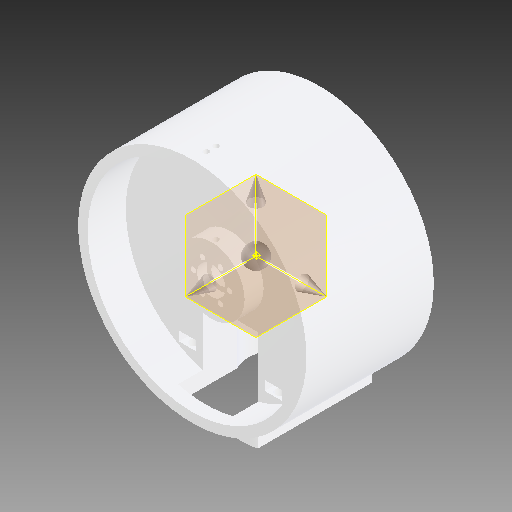
# Autodesk Inventor part: AA035
Saved by Autodesk Inventor 2017 SP1 (Build 210196100, 196)
## iProperties
Created: 2017-10-23
Part Number: AA035
Material: ABS Plastic
Document SubType Name: Modeling
Designer: Zach
Categories: <?xml version="1.0" encoding="UTF-16"?> <MemberInstance><Categories><FamilyTemplate><FamilyTemplateParameter ValueType="xs:double" Id="1" ObjectReferenceKey="da_z" ObjectType="kUserParameterObject"/><FamilyTemplateParameter ValueType="xs:double" Id="2" ObjectReferenceKey="da_b" ObjectType="kUserParameterObject"/><FamilyTemplateParameter ValueType="xs:double" Id="3" ObjectReferenceKey="da_beta" ObjectType="kUserParameterObject"/><FamilyTemplateParameter ValueType="xs:double" Id="4" ObjectReferenceKey="da_da" ObjectType="kUserParameterObject"/><FamilyTemplateParameter ValueType="xs:double" Id="5" ObjectReferenceKey="da_aw" ObjectType="kUserParameterObject"/><FamilyTemplateParameter ValueType="xs:string" Id="6" ObjectReferenceKey="EAIAABAAAACIAQAAAAAAAIAAAAAAAAAA" ObjectType="83910656" SubObjectId="SurfaceGeometry"/></FamilyTemplate><ParamToTemplateMap><ParamToTemplate CategoryParameter="//CategoryParameter[@InternalName='046C89C9-8512-4d59-83FE-43B91F4F132A']" TemplateParameter="1"/><ParamToTemplate CategoryParameter="//CategoryParameter[@InternalName='2552DF32-E462-4b46-AEBF-C6C7768E72AC']" TemplateParameter="2"/><ParamToTemplate CategoryParameter="//CategoryParameter[@InternalName='C9EE641D-15FC-4fae-A226-E94C4372FDD7']" TemplateParameter="3"/><ParamToTemplate><ParamToTemplate CategoryParameter="//CategoryParameter[@InternalName='00B6519A-459B-49c7-AD84-2E56D39A5744']" ConstantValue="0.341447"/></ParamToTemplate><ParamToTemplate><ParamToTemplate CategoryParameter="//CategoryParameter[@InternalName='04B31F0E-C7A6-4894-AA32-9629BEFACF47']" ConstantValue="1.000000"/></ParamToTemplate><ParamToTemplate><ParamToTemplate CategoryParameter="//CategoryParameter[@InternalName='43CBEC2E-7847-49e7-A936-2F7889FCB2D9']" ConstantValue="0.250000"/></ParamToTemplate><ParamToTemplate><ParamToTemplate CategoryParameter="//CategoryParameter[@InternalName='B1EFC894-105D-4ebd-86BF-FA20ED196853']" ConstantValue="0.350000"/></ParamToTemplate><ParamToTemplate><ParamToTemplate CategoryParameter="//CategoryParameter[@InternalName='51175063-3D10-4879-93E8-6246FE8B403D']" ConstantValue="2060000000.000000"/></ParamToTemplate><ParamToTemplate><ParamToTemplate CategoryParameter="//CategoryParameter[@InternalName='A3A52E27-4454-46a9-B0BD-C932399B70AF']" ConstantValue="0.300000"/></ParamToTemplate><ParamToTemplate><ParamToTemplate CategoryParameter="//CategoryParameter[@InternalName='91B76062-C214-41d9-B1B9-14D2AB99603D']" ConstantValue="0.200000"/></ParamToTemplate><ParamToTemplate><ParamToTemplate CategoryParameter="//CategoryParameter[@InternalName='374E806E-8B8A-4dda-A9AA-1039D6500AD2']" ConstantValue="5.000000"/></ParamToTemplate><ParamToTemplate><ParamToTemplate CategoryParameter="//CategoryParameter[@InternalName='2D373A89-B862-43d6-8D0B-0CBF12AB9F6C']" ConstantValue="0.392699"/></ParamToTemplate><ParamToTemplate CategoryParameter="//CategoryParameter[@InternalName='37777632-D6A2-4fac-9D53-DB8ACD95C989']" TemplateParameter="4"/><ParamToTemplate CategoryParameter="//CategoryParameter[@InternalName='FD1017F1-B727-4f7e-9707-0F86F1FF9423']" TemplateParameter="5"/><ParamToTemplate><ParamToTemplate CategoryParameter="//CategoryParameter[@InternalName='9E1B4470-B2D3-4ff1-B813-535BB4CDF51A']" ConstantValue="3520000.000000"/></ParamToTemplate><ParamToTemplate><ParamToTemplate CategoryParameter="//CategoryParameter[@InternalName='F8452263-BFF6-458c-9FB1-07C4B99E95CD']" ConstantValue="11400000.000000"/></ParamToTemplate><ParamToTemplate><ParamToTemplate CategoryParameter="//CategoryParameter[@InternalName='3E3BB259-FD49-497f-8171-6EBC954A3479']" ConstantValue="2.000000"/></ParamToTemplate><ParamToTemplate CategoryParameter="//CategoryParameter[@InternalName='27C3BAF2-7550-4e4b-AE2C-0DB134B7D9B7']" TemplateParameter="6"/></ParamToTemplateMap><Category DisplayName="Gear" InternalName="DC85795E-93AB-48d5-8EEE-5A27447B64BD" Mnemonic="Gear"><CategoryParameter DisplayName="z" InternalName="046C89C9-8512-4d59-83FE-43B91F4F132A" Mnemonic="z"/><CategoryParameter DisplayName="b" InternalName="2552DF32-E462-4b46-AEBF-C6C7768E72AC" Mnemonic="b"/><CategoryParameter DisplayName="||b|" InternalName="C9EE641D-15FC-4fae-A226-E94C4372FDD7" Mnemonic="beta"/><CategoryParameter DisplayName="x" InternalName="00B6519A-459B-49c7-AD84-2E56D39A5744" Mnemonic="x"/><CategoryParameter DisplayName="a*" InternalName="04B31F0E-C7A6-4894-AA32-9629BEFACF47" Mnemonic="a"/><CategoryParameter DisplayName="c*" InternalName="43CBEC2E-7847-49e7-A936-2F7889FCB2D9" Mnemonic="c"/><CategoryParameter DisplayName="r|.f|*" InternalName="B1EFC894-105D-4ebd-86BF-FA20ED196853" Mnemonic="rf"/><CategoryParameter DisplayName="E" InternalName="51175063-3D10-4879-93E8-6246FE8B403D" Mnemonic="E"/><CategoryParameter DisplayName="||m|" InternalName="A3A52E27-4454-46a9-B0BD-C932399B70AF" Mnemonic="mi"/><Category DisplayName="SpurGear" InternalName="26C5A22E-A91E-4dfd-A3B3-23CCAFAE1764" Mnemonic="SpurGear"><CategoryParameter DisplayName="m" InternalName="91B76062-C214-41d9-B1B9-14D2AB99603D" Mnemonic="m"/><CategoryParameter DisplayName="P" InternalName="374E806E-8B8A-4dda-A9AA-1039D6500AD2" Mnemonic="PP"/><CategoryParameter DisplayName="||a|" InternalName="2D373A89-B862-43d6-8D0B-0CBF12AB9F6C" Mnemonic="alpha"/><CategoryParameter DisplayName="d|.a|" InternalName="37777632-D6A2-4fac-9D53-DB8ACD95C989" Mnemonic="da"/><CategoryParameter DisplayName="a|.w|" InternalName="FD1017F1-B727-4f7e-9707-0F86F1FF9423" Mnemonic="aw"/><CategoryParameter DisplayName="||s||.Flim|" InternalName="9E1B4470-B2D3-4ff1-B813-535BB4CDF51A" Mnemonic="sFlim"/><CategoryParameter DisplayName="||s||.Hlim|" InternalName="F8452263-BFF6-458c-9FB1-07C4B99E95CD" Mnemonic="sHlim"/><CategoryParameter DisplayName="type" InternalName="3E3BB259-FD49-497f-8171-6EBC954A3479" Mnemonic="type"/><CategoryParameter DisplayName="PitchDiameter" InternalName="27C3BAF2-7550-4e4b-AE2C-0DB134B7D9B7" Mnemonic="IDS_PITCHDIAM"/></Category></Category></Categories></MemberInstance>
Density: 1.06 g/cm^3
Appearance: CR White
CustomPartVersion: 1
Author: Zach
Title: AA035.ipt
Autodesk Inventor part; units mm, degrees
ref_plane "YZ Plane" through (0, 0, 0) normal (1, 0, 0) x (0, 1, 0)
sketch "Sketch3" plane through (0, 0, 0) normal (0, 0, 1) x (1, 0, 0)
  circle A0 centre (0, 0) radius 60
  dimension "d49" = 120
  constraints: 1 centre point, 1 coincident
  measures "d49" diameter of A0
sketch "Sketch3 outline for Extrusion2" plane through (0, 0, 0) normal (0, 0, 1) x (1, 0, 0)
  circle A0 centre (0, 0) radius 60
extrude "Extrusion2" add sketch "Sketch3 outline for Extrusion2" along normal blind 67
sketch "Sketch4" plane through (0, 0, 0) normal (0, 0, -1) x (-1, 0, 0)
  circle A0 centre (0, 0) radius 5
  dimension "d52" = 10
  constraints: 1 centre point, 1 coincident
  measures "d52" diameter of A0
sketch "Sketch4 outline for Extrusion3" plane through (0, 0, 0) normal (0, 0, -1) x (-1, 0, 0)
  circle A0 centre (0, 0) radius 5
extrude "Extrusion3" cut sketch "Sketch4 outline for Extrusion3" against normal through all
ref_plane "Work Plane11" through (0, 0, 46) normal (0, 0, 1) x (1, 0, 0)
sketch "Sketch6" plane through (0, 0, 46) normal (0, 0, 1) x (1, 0, 0)
  line L0 (-27.5, -53.326823) -> (27.5, -53.326823)
  line L1 (27.5, -53.326823) -> (27.5, -61.326823)
  line L2 (27.5, -61.326823) -> (-27.5, -61.326823)
  line L3 (-27.5, -61.326823) -> (-27.5, -53.326823)
  circle A0 centre (0, 0) radius 5 construction
  circle A1 centre (0, 0) radius 60 construction
  dimension "d63" = 55
  dimension "d64" = 8
  constraints: 8 end point, 2 parallel, 2 point on circle, 1 horizontal, 1 perpendicular
  measures "d63" distance of L1.end L2.end
  measures "d64" distance of L0.end L1.end
sketch "Sketch6 outline for Extrusion5" plane through (0, 0, 46) normal (0, 0, 1) x (1, 0, 0)
  line L0 (-27.5, -53.326823) -> (27.5, -53.326823)
  line L1 (27.5, -53.326823) -> (27.5, -61.326823)
  line L2 (27.5, -61.326823) -> (-27.5, -61.326823)
  line L3 (-27.5, -61.326823) -> (-27.5, -53.326823)
extrude "Extrusion5" add sketch "Sketch6 outline for Extrusion5" along normal mid plane 42
sketch "Sketch7" plane through (0, 0, 46) normal (0, 0, 1) x (1, 0, 0)
  line L0 (-41, -61.326823) -> (41, -61.326823)
  line L1 (41.521509, -76.326823) -> (-41.521509, -76.326823)
  line L2 (27.5, -61.326823) -> (-27.5, -61.326823)
  line L3 (-41.521509, -76.326823) -> (-41, -61.326823)
  line L4 (41.521509, -76.326823) -> (41, -61.326823)
  point P0 (0, 0)
  point P1 (0, -61.326823)
  point P2 (0, -76.326823)
  dimension "d67" = 83.04302
  dimension "d99" = 82
  dimension "d100" = 15
  constraints: 8 end point, 3 midpoint, 1 horizontal, 1 parallel, 1 vertical alignment
  measures "d67" distance of L1.start L1.end
  measures "d99" distance of L0.start L0.end
  measures "d100" distance between parallel lines of L0 L1
sketch "Sketch7 outline for Extrusion6" plane through (0, 0, 46) normal (0, 0, 1) x (1, 0, 0)
  line L0 (-41, -61.326823) -> (0, -61.326823)
  line L1 (0, -61.326823) -> (41, -61.326823)
  line L2 (41, -61.326823) -> (41.521509, -76.326823)
  line L3 (41.521509, -76.326823) -> (-41.521509, -76.326823)
  line L4 (-41.521509, -76.326823) -> (-41, -61.326823)
extrude "Extrusion6" add sketch "Sketch7 outline for Extrusion6" along normal mid plane 80
sketch "Sketch8" plane through (-41.521509, -76.326823, 86) normal (0, -1, 0) x (1, 0, 0)
  line L0 (64.021509, -62.5) -> (19.021509, -62.5) construction
  line L1 (19.021509, -62.5) -> (19.021509, -17.5) construction
  line L2 (19.021509, -17.5) -> (64.021509, -17.5) construction
  line L3 (64.021509, -17.5) -> (64.021509, -62.5) construction
  circle A0 centre (64.021509, -62.5) radius 2.5
  circle A1 centre (64.021509, -17.5) radius 2.5
  circle A2 centre (19.021509, -62.5) radius 2.5
  circle A3 centre (19.021509, -17.5) radius 2.5
  line L4 (0, 0) -> (83.043018, 0)
  line L5 (83.043018, 0) -> (83.043018, -80)
  point P0 (23.25, -86)
  point P1 (41.521509, -17.5)
  point P2 (41.521509, 0)
  point P3 (83.043018, -40)
  dimension "d75" = 45
  dimension "d78" = 5
  dimension "d79" = 5
  dimension "d101" = 45
  dimension "d102" = 5
  dimension "d103" = 5
  dimension "d184" = 17.5
  constraints: 8 end point, 4 centre point, 4 coincident, 3 midpoint, 2 parallel, 1 horizontal, 1 perpendicular, 1 vertical alignment
  measures "d75" distance of L0.end L1.end
  measures "d78" diameter of A2
  measures "d79" diameter of A3
  measures "d101" distance of L1.end L2.end
  measures "d102" diameter of A1
  measures "d103" diameter of A0
  measures "d184" distance between parallel lines of L4 L2
sketch "Sketch8 outline for Extrusion7" plane through (-41.521509, -76.326823, 86) normal (0, -1, 0) x (1, 0, 0)
  circle A0 centre (64.021509, -17.5) radius 2.5
  circle A1 centre (19.021509, -17.5) radius 2.5
extrude "Extrusion7" cut sketch "Sketch8 outline for Extrusion7" against normal blind 25
sketch "Sketch9" plane through (-41.521509, -76.326823, 86) normal (0, -1, 0) x (1, 0, 0)
  circle A0 centre (41.521509, -40) radius 16.5
  circle A1 centre (64.021509, -17.5) radius 2.5 construction
  circle A2 centre (19.021509, -17.5) radius 2.5 construction
  line L0 (83.043018, 0) -> (83.043018, -80) construction
  line L1 (0, 0) -> (83.043018, 0) construction
  line L2 (0, 0) -> (0, -80) construction
  line L3 (83.043018, -80) -> (0, -80) construction
  point P0 (23.25, -86)
  point P1 (0, -40)
  point P2 (41.521509, 0)
  dimension "d82" = 33
  constraints: 2 midpoint, 1 centre point, 1 horizontal alignment, 1 vertical alignment
  measures "d82" diameter of A0
sketch "Sketch9 outline for Extrusion8" plane through (-41.521509, -76.326823, 86) normal (0, -1, 0) x (1, 0, 0)
  circle A0 centre (41.521509, -40) radius 16.5
extrude "Extrusion8" cut sketch "Sketch9 outline for Extrusion8" against normal blind 45
sketch "Sketch14" plane through (0, 0, 46) normal (0, 0, 1) x (1, 0, 0)
  line L0 (16.5, -76.326823) -> (16.5, -31.326823)
  line L1 (16.5, -31.326823) -> (-16.5, -31.326823)
  line L2 (-16.5, -31.326823) -> (-16.5, -16.326823)
  line L3 (-16.5, -16.326823) -> (16.5, -16.326823)
  line L4 (16.5, -16.326823) -> (16.5, -31.326823)
  point P0 (0, 0)
  dimension "d91" = 33
  dimension "d92" = 15
  constraints: 8 end point, 2 parallel, 1 horizontal, 1 perpendicular
  measures "d91" distance of L2.end L3.end
  measures "d92" distance of L1.end L2.end
sketch "Sketch14 outline for Extrusion10" plane through (0, 0, 46) normal (0, 0, 1) x (1, 0, 0)
  line L0 (16.5, -31.326823) -> (-16.5, -31.326823)
  line L1 (-16.5, -31.326823) -> (-16.5, -16.326823)
  line L2 (-16.5, -16.326823) -> (16.5, -16.326823)
  line L3 (16.5, -16.326823) -> (16.5, -31.326823)
extrude "Extrusion10" cut sketch "Sketch14 outline for Extrusion10" along normal mid plane 33
fillet "Fillet4" radius 20 4 edges at (41.2608, -68.8268, 86) (41.2608, -68.8268, 6) (-41.2608, -68.8268, 86) (-41.2608, -68.8268, 6)
ref_plane "Work Plane15" through (0, 0, 25) normal (0, 0, -1) x (-0.9685832, -0.2486899, 0)
sketch "Sketch16" plane through (0, 0, 25) normal (0, 0, -1) x (-0.9685832, -0.2486899, 0)
  circle A0 centre (0, 0) radius 60
  circle A1 centre (0, 0) radius 63
  dimension "d107" = 3
  constraints: 2 centre point
  measures "d107" radial gap between concentric circles of A0 A1
sketch "Sketch16 outline for Extrusion12" plane through (0, 0, 25) normal (0, 0, -1) x (-0.9685832, -0.2486899, 0)
  circle A0 centre (0, 0) radius 63
extrude "Extrusion12" cut sketch "Sketch16 outline for Extrusion12" along normal through all
sketch "Sketch17" plane through (0, 0, 25) normal (0, 0, -1) x (-1, 0, 0)
  circle A0 centre (33.807404, 9.058667) radius 2.5
  circle A1 centre (9.058667, 33.807404) radius 2.5
  circle A2 centre (-24.748737, 24.748737) radius 2.5
  circle A3 centre (-33.807404, -9.058667) radius 2.5
  circle A4 centre (-9.058667, -33.807404) radius 2.5
  circle A5 centre (24.748737, -24.748737) radius 2.5
  line L0 (33.807404, 9.058667) -> (-33.807404, -9.058667) construction
  line L1 (-1.798057, -79.48798) -> (39.754961, -68.353883)
  line L2 (0, 0) -> (32.565454, 0)
  circle A6 centre (0, 0) radius 5
  line L3 (14.422928, -61.326823) -> (27.5, -61.326823)
  line L4 (27.5, -61.326823) -> (27.5, -53.326823)
  arc A7 (27.5, -53.326823) -> (-27.5, -53.326823) centre (0, 0) ccw
  line L5 (-27.5, -53.326823) -> (-27.5, -61.326823)
  line L6 (-27.5, -61.326823) -> (-14.422928, -61.326823)
  arc A8 (-14.422928, -61.326823) -> (14.422928, -61.326823) centre (0, 0) ccw
  dimension "d108" = 5
  dimension "d109" = 35
  dimension "d112" = 360
  dimension "d207" = 15
  constraints: 6 centre point, 6 end point, 1 coincident, 1 horizontal, 1 midpoint, 1 parallel, 13 other
  measures "d108" diameter of A0
  measures "d109" distance of L2.start L0.start
  measures "d207" angle of L0 L2
sketch "Sketch17 outline for Extrusion13" plane through (0, 0, 25) normal (0, 0, -1) x (-1, 0, 0)
  circle A0 centre (33.807404, 9.058667) radius 2.5
  circle A1 centre (9.058667, 33.807404) radius 2.5
  circle A2 centre (-24.748737, 24.748737) radius 2.5
  circle A3 centre (-33.807404, -9.058667) radius 2.5
extrude "Extrusion13" cut sketch "Sketch17 outline for Extrusion13" against normal blind 25
sketch "Sketch20" plane through (0, 0, 67) normal (0, 0, 1) x (1, 0, 0)
  arc A0 (27.5, -53.326823) -> (-27.5, -53.326823) centre (0, 0) ccw
  circle A1 centre (0, 0) radius 60
  circle A2 centre (0, 0) radius 5
  constraints: 1 coincident, 3 other
sketch "Sketch20 outline for Extrusion15" plane through (0, 0, 67) normal (0, 0, 1) x (1, 0, 0)
  circle A0 centre (0, 0) radius 60
  circle A1 centre (0, 0) radius 5
extrude "Extrusion15" add sketch "Sketch20 outline for Extrusion15" along normal blind 25
sketch "Sketch21" plane through (-21.509425, -76.326823, 6) normal (0, -1, 0) x (1, 0, 0)
  line L0 (36.009425, 79) -> (7.009425, 79)
  line L1 (7.009425, 79) -> (7.009425, 55)
  line L2 (7.009425, 55) -> (36.009425, 55)
  line L3 (36.009425, 55) -> (36.009425, 79)
  circle A0 centre (21.509425, 40) radius 16.5
  line L4 (36.009425, 67) -> (7.009425, 67)
  point P0 (21.509425, -6)
  point P1 (21.509425, 67)
  dimension "d124" = 29
  dimension "d125" = 24
  dimension "d126" = 27
  constraints: 10 end point, 3 midpoint, 2 parallel, 1 horizontal, 1 perpendicular, 1 vertical alignment
  measures "d124" distance of L2.end L1.end
  measures "d125" distance of L1.end L0.end
  measures "d126" distance from line of L4 A0.centre
sketch "Sketch21 outline for Extrusion16" plane through (-21.509425, -76.326823, 6) normal (0, -1, 0) x (1, 0, 0)
  line L0 (7.009425, 55) -> (36.009425, 55)
  line L1 (36.009425, 55) -> (36.009425, 79)
  line L2 (36.009425, 79) -> (7.009425, 79)
  line L3 (7.009425, 79) -> (7.009425, 55)
extrude "Extrusion16" cut sketch "Sketch21 outline for Extrusion16" against normal blind 15
sketch "Sketch22" plane through (-27.5, -61.326823, 67) normal (0, 1, 0) x (1, 0, 0)
  line L0 (55, 0) -> (55, 42)
  line L1 (0, 0) -> (0, 42)
  line L2 (0, 0) -> (3, 0)
  line L3 (55, 0) -> (55, -17.911477)
  line L4 (0, 0) -> (0, -17.911477)
  line L5 (5.990575, -19) -> (6.512084, -19) construction
  line L6 (-13.5, 1) -> (-14.021509, 1) construction
  circle A0 centre (5, -1.5) radius 2.5
  line L7 (42, -18) -> (42, 6)
  line L8 (13, -18) -> (42, -18)
  line L9 (13, 6) -> (13, -18)
  line L10 (7, 0) -> (13, 0)
  line L11 (13, 0) -> (13, -18)
  line L12 (13, -18) -> (42, -18)
  line L13 (55, 0) -> (52, 0)
  circle A1 centre (50, -1.5) radius 2.5
  line L14 (48, 0) -> (42, 0)
  line L15 (42, 0) -> (42, -18)
  arc A2 (48, 0) -> (52, 0) centre (50, -1.5) ccw
  arc A3 (3, 0) -> (7, 0) centre (5, -1.5) ccw
  line L16 (5.990575, -19) -> (6.285813, -19)
  line L17 (-13.5, 1) -> (-14.021509, 1)
  line L18 (5.990575, -19) -> (6.512084, -19)
  line L19 (48.487916, -19) -> (49.009425, -19)
  arc A4 (0, -17.911477) -> (6.285813, -19) centre (6.512084, 1) ccw
  arc A5 (48.487916, -19) -> (55, -17.911477) centre (48.487997, 1.023032) ccw
  line L20 (48.487916, -19) -> (6.285813, -19)
  line L21 (5.990575, -19) -> (49.009425, -19)
  ellipse E0 centre (5.990575, 1) end of major axis (-14.021509, 1) minor radius 20 (-14.021509, 1) -> (5.990575, -19) ccw
  line L22 (5.990575, -19) -> (6.512084, -19)
  ellipse E1 centre (6.512084, 1) end of major axis (-13.5, 1) minor radius 20 (-13.5, 1) -> (6.512084, -19) ccw
  line L23 (-13.5, 1) -> (-14.021509, 1)
  ellipse E2 centre (48.487916, 1) end of major axis (68.5, 1) minor radius 20 (48.487916, -19) -> (68.5, 1) ccw
  line L24 (48.487916, -19) -> (49.009425, -19)
  ellipse E3 centre (49.009425, 1) end of major axis (69.021509, 1) minor radius 20 (49.009425, -19) -> (69.021509, 1) ccw
  line L25 (69.021509, 1) -> (68.5, 1)
  point P0 (27.5, 67)
  point P1 (51.789134, -18.726001)
  constraints: 22 end point, 11 point on circle, 4 centre point, 4 point on line, 3 perpendicular, 2 coincident, 2 collinear, 2 vertical, 1 horizontal, 1 horizontal alignment, 10 other
sketch "Sketch22 outline for Extrusion17" plane through (-27.5, -61.326823, 67) normal (0, 1, 0) x (1, 0, 0)
  line L0 (55, -17.911477) -> (55, 0)
  arc A0 (51.789134, -18.726001) -> (55, -17.911477) centre (48.487997, 1.023032) ccw
  arc A1 (48.487916, -19) -> (51.789134, -18.726001) centre (48.487997, 1.023032) ccw
  line L1 (6.285813, -19) -> (48.487916, -19)
  arc A2 (0, -17.911477) -> (6.285813, -19) centre (6.512084, 1) ccw
  line L2 (0, 0) -> (0, -17.911477)
  line L3 (3, 0) -> (0, 0)
  arc A3 (7, 0) -> (3, 0) centre (5, -1.5) cw
  line L4 (13, 0) -> (7, 0)
  line L5 (13, -18) -> (13, 0)
  line L6 (42, -18) -> (13, -18)
  line L7 (42, 0) -> (42, -18)
  line L8 (48, 0) -> (42, 0)
  arc A4 (52, 0) -> (48, 0) centre (50, -1.5) cw
  line L9 (55, 0) -> (52, 0)
extrude "Extrusion17" add sketch "Sketch22 outline for Extrusion17" along normal blind 15
sketch "Sketch23" plane through (-21.509425, -76.326823, 6) normal (0, -1, 0) x (1, 0, 0)
  line L0 (36.009425, 79) -> (36.009425, 55)
  line L1 (36.009425, 55) -> (7.009425, 55)
  line L2 (7.009425, 55) -> (7.009425, 79)
  line L3 (7.009425, 79) -> (36.009425, 79)
  point P0 (21.509425, -6)
sketch "Sketch23 outline for Extrusion18" plane through (-21.509425, -76.326823, 6) normal (0, -1, 0) x (1, 0, 0)
  line L0 (36.009425, 79) -> (36.009425, 55)
  line L1 (36.009425, 55) -> (7.009425, 55)
  line L2 (7.009425, 55) -> (7.009425, 79)
  line L3 (7.009425, 79) -> (36.009425, 79)
extrude "Extrusion18" cut sketch "Sketch23 outline for Extrusion18" against normal blind 20
sketch "Sketch25" plane through (-21.509425, -56.326823, 6) normal (0, -1, 0) x (1, 0, 0)
  line L0 (36.009425, 55) -> (28.383288, 55)
  arc A0 (21.509425, 56.5) -> (5.009425, 40) centre (21.509425, 40) ccw
  line L1 (36.009425, 55) -> (7.009425, 55)
  line L2 (7.009425, 55) -> (7.009425, 47.874008)
  line L3 (7.009425, 47.874008) -> (36.009425, 47.874008)
  line L4 (36.009425, 47.874008) -> (36.009425, 55)
  point P0 (21.509425, -6)
  constraints: 8 end point, 2 parallel, 1 horizontal, 1 perpendicular, 1 point on circle, 1 vertical alignment
sketch "Sketch25 outline for Extrusion20" plane through (-21.509425, -56.326823, 6) normal (0, -1, 0) x (1, 0, 0)
  line L0 (36.009425, 47.874008) -> (36.009425, 55)
  line L1 (7.009425, 47.874008) -> (36.009425, 47.874008)
  line L2 (7.009425, 55) -> (7.009425, 47.874008)
  line L3 (36.009425, 55) -> (7.009425, 55)
extrude "Extrusion20" cut sketch "Sketch25 outline for Extrusion20" along normal blind 25
sketch "Sketch26" plane through (0, 0, 92) normal (0, 0, 1) x (1, 0, 0)
  circle A0 centre (0, 0) radius 5 projected
  circle A1 centre (0, 0) radius 13.5
  dimension "d138" = 27
  constraints: 1 centre point, 1 coincident
  measures "d138" diameter of A1
sketch "Sketch26 outline for Extrusion21" plane through (0, 0, 92) normal (0, 0, 1) x (1, 0, 0)
  circle A0 centre (0, 0) radius 13.5
  circle A1 centre (0, 0) radius 5
extrude "Extrusion21" cut sketch "Sketch26 outline for Extrusion21" against normal blind 10
sketch "Sketch27" plane through (0, 0, 82) normal (0, 0, 1) x (1, 0, 0)
  circle A0 centre (9.525, 0) radius 1.5
  circle A1 centre (4.7625, 8.248892) radius 1.5
  circle A2 centre (-4.7625, 8.248892) radius 1.5
  circle A3 centre (-9.525, 0) radius 1.5
  circle A4 centre (-4.7625, -8.248892) radius 1.5
  circle A5 centre (4.7625, -8.248892) radius 1.5
  point P0 (0, 0)
  dimension "d141" = 3
  dimension "d142" = 9.525
  dimension "d145" = 360
  constraints: 6 centre point, 1 horizontal alignment, 13 other
  measures "d141" diameter of A0
  measures "d142" distance of point (0, 0) A0.centre
sketch "Sketch27 outline for Extrusion22" plane through (0, 0, 82) normal (0, 0, 1) x (1, 0, 0)
  circle A0 centre (9.525, 0) radius 1.5
  circle A1 centre (4.7625, 8.248892) radius 1.5
  circle A2 centre (-4.7625, 8.248892) radius 1.5
  circle A3 centre (-9.525, 0) radius 1.5
  circle A4 centre (-4.7625, -8.248892) radius 1.5
  circle A5 centre (4.7625, -8.248892) radius 1.5
extrude "Extrusion22" cut sketch "Sketch27 outline for Extrusion22" against normal blind 15
sketch "Sketch28" plane through (0, 0, 0) normal (0, 1, 0) x (-1, 0, 0)
  circle A0 centre (0, 79.65) radius 1.5
  circle A1 centre (0, 84.75) radius 1.5
  line L0 (5, 82) -> (-5, 82) projected
  line L1 (0, 82) -> (0, 83.25)
  line L2 (0, 83.25) -> (0, 81.15)
  point P0 (0, 0)
  point P1 (0, 86.25)
  dimension "d151" = 3
  dimension "d150" = 3
  dimension "d153" = 1.25
  dimension "d166" = 2.1
  constraints: 4 end point, 4 vertical alignment, 2 point on circle, 2 vertical, 1 centre point, 1 midpoint, 2 other
  measures "d150" diameter of A1
  measures "d153" distance of L1.start L1.end
  measures "d166" distance of L1.end L2.end
sketch "Sketch28 outline for Extrusion23" plane through (0, 0, 0) normal (0, 1, 0) x (-1, 0, 0)
  circle A0 centre (0, 79.65) radius 1.5
  circle A1 centre (0, 84.75) radius 1.5
extrude "Extrusion23" cut sketch "Sketch28 outline for Extrusion23" along normal through all
sketch "Sketch29" plane through (0, 0, 92) normal (0, 0, 1) x (1, 0, 0)
  circle A0 centre (0, 0) radius 17.5
  circle A1 centre (0, 0) radius 55
  circle A2 centre (0, 0) radius 60 construction
  dimension "d156" = 35
  dimension "d179" = 5
  constraints: 2 centre point, 2 coincident
  measures "d156" diameter of A0
  measures "d179" radial gap between concentric circles of A1 A2
sketch "Sketch29 outline for Extrusion24" plane through (0, 0, 92) normal (0, 0, 1) x (1, 0, 0)
  circle A0 centre (0, 0) radius 55
  circle A1 centre (0, 0) radius 17.5
extrude "Extrusion24" cut sketch "Sketch29 outline for Extrusion24" against normal blind 20
sketch "Sketch30" plane through (0, 0, 82) normal (0, 0, 1) x (1, 0, 0)
  circle A0 centre (0, 0) radius 17.5 projected
sketch "Sketch30 outline for Extrusion25" plane through (0, 0, 82) normal (0, 0, 1) x (1, 0, 0)
  circle A0 centre (0, 0) radius 17.5
extrude "Extrusion25" cut sketch "Sketch30 outline for Extrusion25" along normal through all
sketch "Sketch32" plane through (0, 0, 82) normal (0, 0, 1) x (1, 0, 0)
  circle A0 centre (0, 0) radius 7.5
  dimension "d162" = 15
  constraints: 1 centre point, 1 coincident
  measures "d162" diameter of A0
sketch "Sketch32 outline for Extrusion26" plane through (0, 0, 82) normal (0, 0, 1) x (1, 0, 0)
  circle A0 centre (0, 0) radius 7.5
extrude "Extrusion26" cut sketch "Sketch32 outline for Extrusion26" against normal blind 5
sketch "Sketch34" plane through (0, 0, 72) normal (0, 0, 1) x (1, 0, 0)
  line L0 (-14.5, -56.326823) -> (-14.5, -76.326823)
  line L1 (-14.5, -56.326823) -> (14.5, -56.326823)
  line L2 (14.5, -56.326823) -> (14.5, -21.326823)
  line L3 (14.5, -21.326823) -> (-14.5, -21.326823)
  line L4 (-14.5, -21.326823) -> (-14.5, -56.326823)
  line L5 (14.5, -76.326823) -> (14.5, -56.326823)
  point P0 (0, 0)
  dimension "d167" = 35
  constraints: 8 end point, 2 parallel, 1 coincident, 1 horizontal, 1 perpendicular
  measures "d167" distance of L1.end L2.end
sketch "Sketch34 outline for Extrusion27" plane through (0, 0, 72) normal (0, 0, 1) x (1, 0, 0)
  line L0 (-14.5, -21.326823) -> (-14.5, -56.326823)
  line L1 (14.5, -21.326823) -> (-14.5, -21.326823)
  line L2 (14.5, -56.326823) -> (14.5, -21.326823)
  line L3 (-14.5, -56.326823) -> (14.5, -56.326823)
extrude "Extrusion27" cut sketch "Sketch34 outline for Extrusion27" along normal blind 13 and the other way blind 20
sketch "Sketch35" plane through (41, -61.326823, 66) normal (0, 1, 0) x (1, 0, 0)
  line L0 (-109.517427, 73.180887) -> (100.55897, 73.180887)
  line L1 (100.55897, 73.180887) -> (100.55897, -75.26578)
  line L2 (100.55897, -75.26578) -> (-109.517427, -75.26578)
  line L3 (-109.517427, -75.26578) -> (-109.517427, 73.180887)
  point P0 (-22.5, 23.5)
  constraints: 8 end point, 2 parallel, 1 horizontal, 1 perpendicular
sketch "Sketch35 outline for Extrusion28" plane through (41, -61.326823, 66) normal (0, 1, 0) x (1, 0, 0)
  line L0 (-109.517427, 73.180887) -> (100.55897, 73.180887)
  line L1 (100.55897, 73.180887) -> (100.55897, -75.26578)
  line L2 (100.55897, -75.26578) -> (-109.517427, -75.26578)
  line L3 (-109.517427, -75.26578) -> (-109.517427, 73.180887)
extrude "Extrusion28" cut sketch "Sketch35 outline for Extrusion28" against normal through all
sketch "Sketch37" plane through (0, 0, 92) normal (0, 0, 1) x (1, 0, 0)
  line L0 (-60, 14.5) -> (-53.054218, 14.5)
  line L1 (-53.054218, 14.5) -> (-53.054218, -14.5)
  line L2 (-53.054218, -14.5) -> (-60, -14.5)
  line L3 (-60, -14.5) -> (-60, 14.5)
  circle A0 centre (0, 0) radius 60 construction
  circle A1 centre (0, 0) radius 55 construction
  circle A2 centre (0, 0) radius 60
  point P0 (-53.054218, 0)
  point P1 (-60, 0)
  dimension "d176" = 29
  constraints: 8 end point, 2 horizontal alignment, 2 midpoint, 2 parallel, 1 horizontal, 1 perpendicular, 3 other
  measures "d176" distance of L0.end L1.end
extrude "Extrusion30" [suppressed]
sketch "Sketch40" plane through (-27.5, -61.326823, 67) normal (0, -1, 0) x (1, 0, 0)
  circle A0 centre (5, 1.5) radius 2.5 projected
  circle A1 centre (50, 1.5) radius 2.5 projected
  point P0 (27.5, -67)
sketch "Sketch40 outline for Extrusion33" plane through (-27.5, -61.326823, 67) normal (0, -1, 0) x (1, 0, 0)
  circle A0 centre (5, 1.5) radius 2.5
  circle A1 centre (50, 1.5) radius 2.5
extrude "Extrusion33" cut sketch "Sketch40 outline for Extrusion33" against normal blind 25
sketch "Sketch41" plane through (0, 0, 72) normal (0, 0, 1) x (1, 0, 0)
  line L0 (-20, -36.326823) -> (-25, -36.326823)
  line L1 (-25, -61.326823) -> (-20, -61.326823)
  line L2 (25, -36.326823) -> (20, -36.326823)
  line L3 (20, -61.326823) -> (25, -61.326823)
  line L4 (-27, -41.326823) -> (-18, -41.326823)
  line L5 (-18, -41.326823) -> (-18, -46.326823)
  line L6 (-18, -46.326823) -> (-27, -46.326823)
  line L7 (-27, -46.326823) -> (-27, -41.326823)
  line L8 (18, -41.326823) -> (27, -41.326823)
  line L9 (27, -41.326823) -> (27, -46.326823)
  line L10 (27, -46.326823) -> (18, -46.326823)
  line L11 (18, -46.326823) -> (18, -41.326823)
  point P0 (0, 0)
  point P1 (-22.5, -41.326823)
  point P2 (-22.5, -36.326823)
  point P3 (22.5, -36.326823)
  point P4 (22.5, -41.326823)
  dimension "d192" = 9
  dimension "d193" = 5
  dimension "d194" = 9
  dimension "d195" = 5
  dimension "d196" = 5
  constraints: 16 end point, 4 midpoint, 4 parallel, 2 horizontal, 2 perpendicular, 2 vertical alignment, 1 horizontal alignment, 1 point on line
  measures "d192" distance of L5.end L6.end
  measures "d193" distance of L4.end L5.end
  measures "d194" distance of L9.end L10.end
  measures "d195" distance of L8.end L9.end
  measures "d196" distance between parallel lines of L4 L0
sketch "Sketch41 outline for Extrusion34" plane through (0, 0, 72) normal (0, 0, 1) x (1, 0, 0)
  line L0 (-27, -41.326823) -> (-18, -41.326823)
  line L1 (-18, -41.326823) -> (-18, -46.326823)
  line L2 (-18, -46.326823) -> (-27, -46.326823)
  line L3 (-27, -46.326823) -> (-27, -41.326823)
  line L4 (18, -41.326823) -> (27, -41.326823)
  line L5 (27, -41.326823) -> (27, -46.326823)
  line L6 (27, -46.326823) -> (18, -46.326823)
  line L7 (18, -46.326823) -> (18, -41.326823)
extrude "Extrusion34" cut sketch "Sketch41 outline for Extrusion34" against normal blind 8.5
sketch "Sketch42" plane through (-27.5, -61.326823, 67) normal (0, -1, 0) x (1, 0, 0)
  circle A0 centre (5, 1.5) radius 2.5 projected
  circle A1 centre (50, 1.5) radius 2.5 projected
  circle A2 centre (5, -38.5) radius 2.5
  circle A3 centre (50, -38.5) radius 2.5
  point P0 (27.5, -67)
  dimension "d199" = 5
  dimension "d200" = 5
  dimension "d201" = 40
  constraints: 2 centre point, 2 vertical alignment, 1 horizontal alignment
  measures "d199" diameter of A2
  measures "d200" diameter of A3
  measures "d201" distance of A2.centre A0.centre
sketch "Sketch42 outline for Extrusion35" plane through (-27.5, -61.326823, 67) normal (0, -1, 0) x (1, 0, 0)
  circle A0 centre (5, -38.5) radius 2.5
  circle A1 centre (50, -38.5) radius 2.5
extrude "Extrusion35" cut sketch "Sketch42 outline for Extrusion35" against normal blind 25
sketch "Sketch43" plane through (0, 0, 25) normal (0, 0, -1) x (-1, 0, 0)
  line L0 (27, -41.326823) -> (18, -41.326823)
  line L1 (27, -46.326823) -> (27, -41.326823)
  line L2 (18, -46.326823) -> (27, -46.326823)
  line L3 (18, -41.326823) -> (18, -46.326823)
  line L4 (-18, -41.326823) -> (-27, -41.326823)
  line L5 (-18, -46.326823) -> (-18, -41.326823)
  line L6 (-27, -46.326823) -> (-18, -46.326823)
  line L7 (-27, -41.326823) -> (-27, -46.326823)
  point P0 (0, 0)
sketch "Sketch43 outline for Extrusion36" plane through (0, 0, 25) normal (0, 0, -1) x (-1, 0, 0)
  line L0 (18, -41.326823) -> (27, -41.326823)
  line L1 (27, -41.326823) -> (27, -46.326823)
  line L2 (27, -46.326823) -> (18, -46.326823)
  line L3 (18, -46.326823) -> (18, -41.326823)
  line L4 (-27, -41.326823) -> (-18, -41.326823)
  line L5 (-18, -41.326823) -> (-18, -46.326823)
  line L6 (-18, -46.326823) -> (-27, -46.326823)
  line L7 (-27, -46.326823) -> (-27, -41.326823)
extrude "Extrusion36" cut sketch "Sketch43 outline for Extrusion36" against normal blind 8.5
equation "\"d43\" = da_aw"
equation "\"d46\" = da_aw"
equation "\"da_aw\" = 81.5"
body "Solid1"
